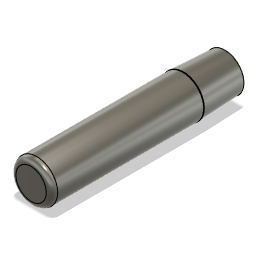
Oak_Cylindrical_Topper (Autodesk Fusion 360 design; units mm, degrees)
Autodesk Fusion 360 part; units mm, degrees
note: some values were not read from the file. Set by a fixed rule: which sketch regions a step uses.
sketch "Sketch1" plane through (0, 0, 0) normal (0, 1, 0) x (1, 0, 0)
  line L0 (0, 0) -> (0, -102)
  line L1 (0, -102) -> (-11, -102)
  line L2 (-11, -102) -> (-11, -22)
  line L3 (-11, -22) -> (-10, 0)
  line L4 (-10, 0) -> (-6, 0)
  line L5 (-6, 0) -> (-6, -102)
  line L6 (-6, -22) -> (0, -22)
  line L7 (-6, -24) -> (0, -24)
  line L8 (-6, -100) -> (0, -100)
  line L9 (-6, -24) -> (-6.6, -24)
  line L10 (-8.6, -26) -> (-8.6, -100)
  line L11 (-8.6, -100) -> (-6, -100)
  arc A0 (-6.6, -24) -> (-8.6, -26) centre (-6.6, -26) ccw
  line L12 (-6.2, -100) -> (-8.6, -97.6)
  dimension "d1" = 102
  dimension "d2" = 6
  dimension "d3" = 5
  dimension "d4" = 4
  dimension "d7" = 22
  dimension "d8" = 80
  dimension "d9" = 2
  dimension "d12" = 2
  dimension "d13" = 2.4
  dimension "d14" = 2
  dimension "d15" = 135
  dimension "d16" = 2.4
  constraint coincident L0.start origin
  constraint vertical L0
  constraint perpendicular L0 L1
  constraint perpendicular L1 L2
  constraint perpendicular L0 L4
  constraint coincident L1 L5.end
  constraint perpendicular L1 L5
  constraint equal L0 L5
  constraint coincident L5 L6.start
  constraint coincident L0 L6.end
  constraint perpendicular L0 L6
  constraint coincident L5 L7.start
  constraint coincident L0 L7.end
  constraint perpendicular L0 L7
  constraint coincident L2.end L6
  constraint coincident L5 L8.start
  constraint coincident L0 L8.end
  constraint parallel L1 L8
  constraint perpendicular L5 L9
  constraint perpendicular L9 L10
  constraint perpendicular L10 L11
  constraint tangent L9 A0
  constraint tangent L10 A0
  constraint coincident L11 L12.start
  constraint coincident L10 L12.end
  measures "d1" distance of L0.start L0.end
  measures "d2" distance of L0.start L4.end
  measures "d3" distance of L2 L5
  measures "d4" distance of L3.end L4.end
  measures "d7" vertical distance of L2.end L3.end
  measures "d8" distance of L1.end L2.end
  measures "d9" distance of L6 L7
  measures "d12" distance of L0.end L8.end
  measures "d13" distance of L2 L10
  measures "d14" radius of A0
  measures "d15" angle of L11 L12
  measures "d16" distance of L10.end L12.start
revolve "Revolve1" add sketch "Sketch1" angle 360 about axis through (0, 0, 0) along (0, 0, 1) contours L0 L5 L6 L7 | L1 L2 L3 L4 L5 L9 L10 L11 A0 | L0 L1 L5 L8 | L10 L11 L12
fillet "Fillet1" radius 3 1 edges at (-10.2556, 3.9778, 102)
fillet "Fillet2" radius 8 1 edges at (-10.2556, 3.9778, 22)
sketch "Sketch2" plane through (0, 0, 0) normal (0, 0, -1) x (-1, 0, 0)
  circle A0 centre (0, 0) radius 10
  circle A1 centre (0, 0) radius 6
  circle A2 centre (0, 6) radius 1.5
  dimension "d21" = 3
  constraint coincident A1 A2.centre
  measures "d21" diameter of A2
extrude "Extrude1" cut sketch "Sketch2" against normal up to surface (22 mm away) contours A1 A2 picked at (0.5033, 6.4154)
fillet "Fillet3" radius 1 2 edges at (-1.4882, 5.8125, 11) (1.4882, 5.8125, 11)
chamfer "Chamfer1" distance 1 angle 45 4 edges at (0, -6, 0) (-1.6849, 5.9022, 0) (0, 7.5, 0) (1.6849, 5.9022, 0)
named bodies: "Oak_Cylindrical_Topper"
